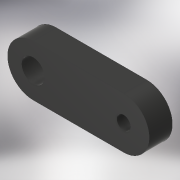
# Autodesk Inventor part: TA07
Saved by Autodesk Inventor 2017 (Build 210142000, 142)
## iProperties
Created: 2019-04-10
Part Number: TA07
Material: ABS Plastic
Document SubType Name: Modeling
Designer: Dell
Density: 1.06 g/cm^3
Appearance: Smooth - Black
Author: Dell
Autodesk Inventor part; units mm, degrees
ref_plane "YZ Plane" through (0, 0, 0) normal (1, 0, 0) x (0, 1, 0)
ref_plane "XZ Plane" through (0, 0, 0) normal (0, 1, 0) x (-1, 0, 0)
ref_plane "XY Plane" through (0, 0, 0) normal (0, 0, 1) x (1, 0, 0)
sketch "Sketch1" plane through (0, 0, 0) normal (0, 0, 1) x (1, 0, 0)
  circle A0 centre (0, 0) radius 2.5
  circle A1 centre (0, 0) radius 5.5
  circle A2 centre (19.5, 0) radius 1.5
  circle A3 centre (19.5, 0) radius 5.5
  line L0 (0, 5.5) -> (19.5, 5.5)
  line L1 (0, -5.5) -> (19.5, -5.5)
  dimension "d0" = 5
  dimension "d1" = 11
  dimension "d2" = 3
  dimension "d3" = 11
  dimension "d4" = 19.5
  constraints: 4 centre point, 4 end point, 4 point on circle, 4 tangent, 3 coincident, 1 horizontal alignment
  measures "d0" diameter of A0
  measures "d1" diameter of A1
  measures "d2" diameter of A2
  measures "d3" diameter of A3
  measures "d4" distance of A2.centre point (0, 0)
extrude "Extrusion1" add sketch "Sketch1" along normal blind 5
body "Solid1"
